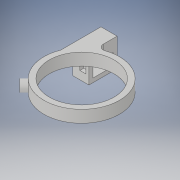
# Autodesk Inventor part: DC_Ring
Saved by Autodesk Inventor 2019 (Build 230136000, 136)
## iProperties
Created: 2019-11-14
Part Number: DC_Ring
Material: Generic
Document SubType Name: Modeling
Designer: James
Density: 1 g/cm^3
Appearance: Default
Author: James
Autodesk Inventor part; units mm, degrees
ref_plane "YZ Plane" through (0, 0, 0) normal (1, 0, 0) x (0, 1, 0)
ref_plane "XZ Plane" through (0, 0, 0) normal (0, 1, 0) x (-1, 0, 0)
sketch "Sketch1" plane through (0, 0, 0) normal (0, 1, 0) x (-1, 0, 0)
  circle A0 centre (0, 0) radius 16.05
  circle A1 centre (0, 0) radius 18.75
  point P0 (18.75, 0)
  point P1 (13.2583, 13.2583)
  dimension "d0" = 32.1
  dimension "d4" = 45
  dimension "d9" = 2.7
  constraints: 2 centre point, 2 coincident, 2 point on circle, 1 horizontal alignment
  measures "d0" diameter of A0
  measures "d9" radial gap between concentric circles of A0 A1
extrude "Extrusion1" add sketch "Sketch1" along normal blind 6
ref_plane "Work Plane1" through (-13.2583, 0, 13.2583) normal (-0.7071, 0, 0.7071) x (0, -1, 0)
sketch "Sketch2" plane through (-13.2583, 0, 13.2583) normal (-0.7071, 0, 0.7071) x (0, -1, 0)
  circle A0 centre (-3, 0) radius 1.5
  circle A1 centre (-3, 0) radius 2.5
  point P0 (0, 0)
  dimension "d5" = 3
  dimension "d6" = 5
  dimension "d7" = 3
  dimension "d10" = 0
  constraints: 2 centre point, 1 coincident
  measures "d5" diameter of A0
  measures "d6" diameter of A1
  measures "d7" distance of point (0, 0) A0.centre
  measures "d10" vertical distance of point (0, 0) A0.centre
extrude "Extrusion2" add sketch "Sketch2" along normal mid plane 6
sketch "Sketch3" plane through (-15.3796, 3, 15.3796) normal (-0.7071, 0, 0.7071) x (0.7071, 0, 0.7071)
  circle A0 centre (0, 0) radius 1.5
  point P0 (0, -3)
  constraints: 1 centre point
extrude "Extrusion3" cut sketch "Sketch3" against normal blind 9.75
sketch "Sketch6" plane through (0, 0, 0) normal (0, -1, 0) x (1, 0, 0)
  line L0 (-17.4129, -27) -> (-9.4129, -27)
  line L1 (-9.4129, -27) -> (-9.4129, -13)
  line L2 (-9.4129, -13) -> (-17.4129, -13)
  line L3 (-17.4129, -13) -> (-17.4129, -27)
  circle A0 centre (0, 0) radius 16.05 projected
  point P0 (-13.4129, -27)
  dimension "d15" = 14
  dimension "d16" = 8
  dimension "d34" = 13
  constraints: 8 end point, 2 parallel, 1 horizontal, 1 midpoint, 1 perpendicular, 2 other
  measures "d15" distance between parallel lines of L0 L2
  measures "d16" distance of L0.start L0.end
  measures "d34" distance from line of point (0, 0) L2
extrude "Extrusion4" add sketch "Sketch6" along normal blind 8 contours L3 L2 L1 L0
sketch "Sketch7" plane through (-17.4129, 0, -27) normal (-1, 0, 0) x (0, 0, 1)
  line L0 (12, 0) -> (2, 0)
  line L1 (2, 0) -> (2, -6)
  line L2 (2, -6) -> (12, -6)
  line L3 (12, -6) -> (12, 0)
  line L4 (14, 0) -> (14, -8) projected
  line L5 (14, -8) -> (0, -8) projected
  point P0 (27, 0)
  dimension "d19" = 10
  dimension "d20" = 6
  dimension "d21" = 2
  dimension "d22" = 2
  constraints: 8 end point, 2 parallel, 1 horizontal, 1 perpendicular
  measures "d19" distance of L1.end L2.end
  measures "d20" distance of L0.end L1.end
  measures "d21" distance between parallel lines of L4 L3
  measures "d22" distance between parallel lines of L5 L2
extrude "Extrusion5" cut sketch "Sketch7" against normal blind 10
sketch "Sketch8" plane through (0, 0, -13) normal (0, 0, 1) x (1, 0, 0)
  line L0 (-13.5116, 0) -> (-9.4129, 0) projected
  line L1 (-10.9129, 0) -> (-13.9129, 0)
  line L2 (-13.9129, 0) -> (-13.9129, -4)
  line L3 (-13.9129, -4) -> (-10.9129, -4)
  line L4 (-10.9129, -4) -> (-10.9129, 0)
  line L5 (-9.4129, 0) -> (-9.4129, -8) projected
  line L6 (-17.4129, -6) -> (-9.4129, -6) projected
  point P0 (0, 0)
  point P1 (-4, 0)
  dimension "d25" = 1.5
  dimension "d26" = 3
  dimension "d27" = 2
  constraints: 8 end point, 2 parallel, 1 horizontal, 1 perpendicular, 1 point on line
  measures "d25" distance between parallel lines of L5 L4
  measures "d26" distance of L2.end L3.end
  measures "d27" distance between parallel lines of L6 L3
extrude "Extrusion6" cut sketch "Sketch8" against normal blind 15.25
sketch "Sketch9" plane through (-9.4129, -8, -27) normal (0, 0, -1) x (-1, 0, 0)
  line L0 (6.6371, 8) -> (-25.4629, 8) projected
  line L1 (0, 8) -> (8, 8)
  line L2 (8, 8) -> (8, 14)
  line L3 (8, 14) -> (0, 14)
  line L4 (0, 14) -> (0, 8)
  point P0 (-9.4129, 8)
  dimension "d30" = 6
  constraints: 8 end point, 3 point on line, 2 parallel, 1 horizontal, 1 perpendicular
  measures "d30" distance of L3.end L1.start
extrude "Extrusion7" add sketch "Sketch9" against normal blind 20.5
sketch "Sketch10" plane through (0, 0, 0) normal (0, -1, 0) x (1, 0, 0)
  circle A0 centre (0, 0) radius 16.05
  arc A1 (-9.4129, -13) -> (-14.6749, -6.5) centre (0, 0) ccw projected
  constraints: 1 centre point, 1 coincident, 1 concentric
extrude "Extrusion8" cut sketch "Sketch10" against normal blind 12.5
fillet "Fillet2" radius 2.5 1 edges at (-9.4129, 3, -16.216)
body "Solid1"
